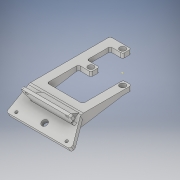
# Autodesk Inventor part: v3burnisher_cameras_mount
Saved by Autodesk Inventor 2019 (Build 230136000, 136)
## iProperties
Created: 2019-11-07
Part Number: v3burnisher_cameras_mount
Material: Generic
Document SubType Name: Modeling
Designer: luua
Density: 1 g/cm^3
Appearance: Default
Author: luua
Autodesk Inventor part; units mm, degrees
sketch "Sketch1" plane through (0, 0, 0) normal (0, 1, 0) x (-1, 0, 0)
  circle A0 centre (-17.6777, 17.6777) radius 3.3
  circle A1 centre (-17.6777, -17.6777) radius 3.25 construction
  circle A2 centre (17.6777, -17.6777) radius 3.3
  circle A3 centre (17.6777, 17.6777) radius 3.25 construction
  circle A4 centre (25, 0) radius 3 construction
  circle A5 centre (0, 0) radius 30.5 construction
  circle A6 centre (0, 0) radius 16.75 construction
  line L0 (36.4277, -22.4277) -> (12.9277, -22.4277)
  line L1 (12.9277, -22.4277) -> (12.9277, -12.9277)
  line L2 (12.9277, -12.9277) -> (26.9277, -12.9277)
  line L3 (26.9277, 57.5) -> (-12.9277, 57.5)
  line L4 (-12.9277, 57.5) -> (-12.9277, 12.3777)
  line L5 (-12.9277, 12.3777) -> (-22.4277, 12.3777)
  line L6 (-22.4277, 12.3777) -> (-22.4277, 67.5)
  line L7 (36.4277, -22.4277) -> (36.4277, 67.5)
  line L8 (32.5, 32.5) -> (-32.5, 32.5) construction
  line L9 (-32.5, 32.5) -> (-32.5, -32.5) construction
  line L10 (-32.5, -32.5) -> (32.5, -32.5) construction
  line L11 (32.5, -32.5) -> (32.5, 32.5) construction
  line L12 (32.5, 32.5) -> (-32.5, -32.5) construction
  line L13 (-32.5, 32.5) -> (32.5, -32.5) construction
  line L14 (20, 32.5) -> (20, 57.5) construction
  line L15 (20, 57.5) -> (-5, 57.5) construction
  line L16 (-5, 57.5) -> (-5, 32.5) construction
  line L17 (5, 57.5) -> (5, 32.5) construction
  line L18 (5, 32.5) -> (-5, 32.5) construction
  line L19 (36.4277, 67.5) -> (-22.4277, 67.5)
  line L20 (26.9277, -12.9277) -> (26.9277, 12.9277)
  line L21 (26.9277, 12.9277) -> (12.9277, 12.9277)
  line L22 (12.9277, 12.9277) -> (12.9277, 22.4277)
  line L23 (12.9277, 22.4277) -> (26.9277, 22.4277)
  circle A7 centre (17.6777, 17.6777) radius 3.25
  line L24 (26.9277, 22.4277) -> (26.9277, 57.5)
  point P0 (0, 32.5)
  point P1 (12.9277, -17.6777)
  point P2 (-17.6777, 12.3777)
  dimension "d0" = 65
  dimension "d1" = 65
  dimension "d2" = 10
  dimension "d3" = 15
  dimension "d4" = 25
  dimension "d5" = 2
  dimension "d7" = 4.75
  dimension "d8" = 4.75
  dimension "d9" = 4.75
  dimension "d96" = 6.6
  dimension "d97" = 6.6
  dimension "d99" = 4.75
  dimension "d100" = 4.75
  dimension "d101" = 9.5
  dimension "d102" = 14
  dimension "d103" = 9.5
  dimension "d104" = 10
  constraints: 50 end point, 10 perpendicular, 8 centre point, 6 midpoint, 5 point on line, 5 vertical, 4 horizontal, 2 collinear, 2 horizontal alignment, 2 parallel, 1 coincident, 1 concentric, 1 vertical alignment, 13 other
  measures "d0" distance of L10.end L9.end
  measures "d1" distance of L9.end L8.end
  measures "d2" distance between parallel lines of L16 L17
  measures "d3" distance between parallel lines of L14 L17
  measures "d4" distance of L15.end L16.end
  measures "d5" distance edge to line of A0 L5
  measures "d7" distance from line of A0.centre L4
  measures "d8" distance from line of L0 A2.centre
  measures "d9" distance from line of A2.centre L1
  measures "d96" diameter of A0
  measures "d97" diameter of A2
  measures "d99" distance from line of L22 A3.centre
  measures "d100" distance from line of L21 A3.centre
  measures "d101" distance between parallel lines of L23 L21
  measures "d102" distance of L1.end L2.end
  measures "d103" distance between parallel lines of L20 L7
  measures "d104" distance between parallel lines of L19 L15
extrude "Extrusion1" add sketch "Sketch1" along normal blind 5
ref_plane "Work Plane1" through (22.4277, 5, 67.5) normal (0, 0.8660254, 0.5) x (1, 0, 0)
sketch "Sketch4" plane through (22.4277, 5, 67.5) normal (0, 0.8660254, 0.5) x (1, 0, 0)
  line L0 (-58.8553, 0) -> (0, 0) projected
  line L1 (-23, 20) -> (-23, 0) construction
  circle A0 centre (-51, -25.748) radius 1.5
  circle A1 centre (5, -25.748) radius 1.5
  circle A2 centre (-23, -21.748) radius 3.25
  line L2 (-51, -25.748) -> (5, -25.748) construction
  line L3 (0, -2.5) -> (-58.8553, -2.5) projected
  line L4 (-58.8553, 77.8796) -> (-58.8553, 0) projected
  line L5 (-58.8553, -2.5) -> (-58.8553, 75.3796) projected
  line L6 (0, 45.2373) -> (0, -2.5) projected
  line L7 (0, 0) -> (0, -2.5)
  line L8 (0, -2.5) -> (12, -25.748)
  line L9 (12, -25.748) -> (12, -27.748)
  line L10 (-56.8553, -29.748) -> (10, -29.748)
  arc A3 (10, -29.748) -> (12, -27.748) centre (10, -27.748) ccw
  line L11 (-58.8553, -2.5) -> (-58.8553, -27.748)
  arc A4 (-58.8553, -27.748) -> (-56.8553, -29.748) centre (-56.8553, -27.748) ccw
  point P0 (-23, -25.748)
  point P1 (12, -29.748)
  dimension "d43" = 3
  dimension "d44" = 6.5
  dimension "d45" = 4
  dimension "d58" = 4
  dimension "d83" = 56
  dimension "d114" = 2
  constraints: 14 end point, 5 centre point, 4 point on circle, 4 tangent, 4 vertical, 3 point on line, 2 horizontal alignment, 2 vertical alignment, 1 coincident, 1 equal radius, 1 horizontal, 1 midpoint, 1 parallel, 1 perpendicular
  measures "d43" diameter of A0
  measures "d44" diameter of A2
  measures "d45" distance from line of L2 A2.centre
  measures "d58" distance from line of L10 L2.start
  measures "d83" distance of A1.centre L2.start
  measures "d114" radius of A4
extrude "Extrusion3" add sketch "Sketch4" against normal blind 5
sketch "Sketch5" plane through (22.4277, 5, 67.5) normal (0, 0.8660254, 0.5) x (1, 0, 0)
  line L0 (-45.5, -8.698) -> (-0.5, -8.698)
  line L1 (-0.5, -8.698) -> (-0.5, -11.698)
  line L2 (-0.5, -11.698) -> (-45.5, -11.698)
  line L3 (-45.5, -11.698) -> (-45.5, -8.698)
  line L4 (-58.8553, 0) -> (0, 0) projected
  line L5 (-58.8553, 0) -> (-58.8553, -27.748) projected
  line L6 (0, -2.5) -> (0, 0) projected
  line L7 (-56.8553, -29.748) -> (10, -29.748) projected
  line L8 (12, -27.748) -> (12, -25.748) projected
  line L9 (12, -25.748) -> (0, -2.5) projected
  arc A0 (10, -29.748) -> (12, -27.748) centre (10, -27.748) ccw projected
  circle A1 centre (-23, -21.748) radius 3.25 projected
  arc A2 (-58.8553, -27.748) -> (-56.8553, -29.748) centre (-56.8553, -27.748) ccw projected
  point P0 (-22.4277, 55.9567)
  point P1 (-23, -11.698)
  dimension "d50" = 3
  dimension "d51" = 45
  dimension "d62" = 10.05
  constraints: 8 end point, 2 parallel, 1 horizontal, 1 midpoint, 1 perpendicular, 1 vertical alignment
  measures "d50" distance of L0.end L1.end
  measures "d51" distance of L0.start L0.end
  measures "d62" distance from line of L2 A1.centre
extrude "Extrusion4" add sketch "Sketch5" along normal blind 4 contours L0 L1 L2 L3
sketch "Sketch7" plane through (22.4277, 8.4641, 69.5) normal (0, 0.8660254, 0.5) x (1, 0, 0)
  line L0 (-0.5, -8.698) -> (-45.5, -8.698) projected
  line L1 (-45.5, -8.698) -> (-45.5, -11.698) projected
  line L2 (-45.5, -11.698) -> (-0.5, -11.698) projected
  line L3 (-0.5, -11.698) -> (-0.5, -8.698) projected
  line L4 (-50.5, -11.698) -> (4.5, -11.698)
  line L5 (4.5, -11.698) -> (4.5, -8.698)
  line L6 (4.5, -8.698) -> (-50.5, -8.698)
  line L7 (-50.5, -8.698) -> (-50.5, -11.698)
  line L8 (-50.5, -11.698) -> (4.5, -8.698) construction
  line L9 (4.5, -11.698) -> (-50.5, -8.698) construction
  point P0 (-23, -10.198)
  dimension "d85" = 55
  constraints: 12 end point, 2 midpoint, 2 parallel, 1 horizontal, 1 perpendicular
  measures "d85" distance of L6.end L5.end
extrude "Extrusion5" add sketch "Sketch7" along normal blind 12
sketch "Sketch6" plane through (-23.0723, -0.849, 77.6307) normal (0, -0.5, 0.8660254) x (1, 0, 0)
  circle A0 centre (0, 12.5) radius 1.6
  circle A1 centre (45, 12.5) radius 1.6
  line L0 (45, 0) -> (0, 0) projected
  line L1 (45, 0) -> (45, 4) projected
  line L2 (0, 0) -> (0, 4) projected
  line L3 (0, 12.5) -> (45, 12.5) construction
  line L4 (45, 4) -> (50, 4) projected
  line L5 (50, 4) -> (50, 16) projected
  line L6 (-5, 16) -> (50, 16) projected
  line L7 (-5, 4) -> (-5, 16) projected
  line L8 (-5, 4) -> (0, 4) projected
  point P0 (22.5, 16)
  point P1 (22.5, 12.5)
  dimension "d67" = 12.5
  dimension "d74" = 3.2
  dimension "d75" = 3.2
  dimension "d84" = 45
  constraints: 2 centre point, 2 end point, 1 horizontal, 1 horizontal alignment, 1 midpoint, 1 vertical alignment
  measures "d67" distance from line of L0 L3.start
  measures "d74" diameter of A0
  measures "d75" diameter of A1
  measures "d84" distance of L3.end L3.start
extrude "Extrusion6" cut sketch "Sketch6" against normal up to next contours A0 | A1
sketch "Sketch8" plane through (-23.0723, -0.849, 77.6307) normal (0, -0.5, 0.8660254) x (1, 0, 0)
  line L0 (-5, 16) -> (50, 16) projected
  line L1 (22.5, 16) -> (22.5, 0) construction
  line L2 (-13.3553, 0) -> (45.5, 0) projected
  line L3 (0, 0) -> (0, 4) projected
  line L4 (0, 4) -> (-5, 4)
  line L5 (-5, 4) -> (-5, 9)
  line L6 (-5, 4) -> (-5, 16) projected
  line L7 (-5, 9) -> (0, 4)
  line L8 (45, 4) -> (50, 4)
  line L9 (50, 4) -> (50, 9)
  line L10 (50, 9) -> (45, 4)
  point P0 (23.0723, -38.0801)
  dimension "d86" = 5
  constraints: 14 end point, 3 symmetric about line, 2 point on line, 1 horizontal, 1 midpoint, 1 vertical
  measures "d86" distance of L4.end L5.end
extrude "Extrusion7" cut sketch "Sketch8" against normal up to surface (3 mm away)
ref_plane "Work Plane2" through (-0.5723, 14.5074, 83.0327) normal (-1, 0, 0) x (0, -0.5, 0.8660254)
sketch "Sketch9" plane through (-0.5723, 14.5074, 83.0327) normal (-1, 0, 0) x (0, -0.5, 0.8660254)
  line L0 (0, -6) -> (-8, -16)
  line L1 (-8, -16) -> (0, -16)
  line L2 (0, -16) -> (0, -6)
  point P0 (-64.6547, -54.0801)
  dimension "d88" = 10
  dimension "d89" = 8
  constraints: 6 end point, 1 horizontal, 1 perpendicular
  measures "d88" distance of L1.end L0.start
  measures "d89" distance of L0.end L1.end
extrude "Extrusion8" add sketch "Sketch9" along normal mid plane 40
ref_plane "Work Plane3" through (-7, 0, 12.3777) normal (1, 0, 0) x (0, 0, -1)
sketch "Sketch10" plane through (-7, 0, 12.3777) normal (1, 0, 0) x (0, 0, -1)
  line L0 (-70.3848, -9.5853) -> (-10.05, 0)
  line L1 (0, 0) -> (-53.7826, 0) projected
  line L2 (-70.3848, -9.5853) -> (-53.7826, 0)
  line L3 (-53.7826, 0) -> (-10.05, 0)
  line L4 (-68.642, -8.5791) -> (-74.2712, -11.8291) projected
  point P0 (-78.3848, -14.2041)
  dimension "d115" = 8
  constraints: 6 end point, 2 point on line, 1 coincident, 1 collinear
  measures "d115" horizontal distance of point (-78.385, -14.204) L0.start
extrude "Extrusion11" add sketch "Sketch10" along normal blind 9.5 from surface at -29.4277
extrude "Extrusion12" add sketch "Sketch10" along normal blind 9.5 from surface at 19.9277
sketch "Sketch12" plane through (12.9277, 0, 57.5) normal (-1, 0, 0) x (0, 0, 1)
  line L0 (8.6603, 0) -> (25.2625, -9.5853) projected
  line L1 (0, 0) -> (0, 5) projected
  line L2 (8.6603, 0) -> (0, 0)
  line L3 (8.6603, 0) -> (25.2625, -9.5853)
  line L4 (32.2984, -7.874) -> (12.1651, 3.75) projected
  line L5 (25.2625, -9.5853) -> (-35.0723, 0) projected
  line L6 (25.2625, -9.5853) -> (0, -5.5719)
  line L7 (0, 0) -> (0, -5.5719)
  point P0 (-57.5, 0)
  constraints: 8 end point, 1 horizontal, 1 parallel, 1 point on line, 1 vertical
extrude "Extrusion13" add sketch "Sketch12" along normal up to next
fillet "Fillet3" [suppressed]
sketch "Sketch13" plane through (22.4277, 0.6699, 65) normal (0, -0.8660254, -0.5) x (1, 0, 0)
  arc A0 (-19.9949, 20.5104) -> (-26.0051, 20.5104) centre (-23, 21.748) ccw projected
  arc A1 (-26.0051, 20.5104) -> (-19.9949, 20.5104) centre (-23, 21.748) ccw projected
  circle A2 centre (-23, 21.748) radius 7.5
  point P0 (-22.4277, -55.9567)
  dimension "d118" = 15
  constraints: 1 centre point, 1 coincident
  measures "d118" diameter of A2
extrude "Extrusion14" cut sketch "Sketch13" along normal blind 10 contours A1 A0
extrude "Extrusion15" cut sketch "Sketch13" along normal blind 5
fillet "Fillet4" radius 2 8 edges at (26.9277, 7.6952, 80.8317) (-28.0723, 7.6952, 80.8317) (-28.0723, 13.7574, 84.3317) (-23.0723, -0.099, 76.3317) (21.9277, -0.099, 76.3317) (26.9277, 13.7574, 84.3317) (-23.0723, 3.3651, 78.3317) (21.9277, 3.3651, 78.3317)
fillet "Fillet4" radius 5 1 edges at (-7, 5, 67.5)
fillet "Fillet4" radius 2 12 edges at (-26.9277, 2.5, 22.4277) (-26.9277, 2.5, 12.9277) (-26.9277, 2.5, -12.9277) (-12.9277, 2.5, -22.4277) (-12.9277, 2.5, -12.9277) (-12.9277, 2.5, 12.9277) (-12.9277, 2.5, 22.4277) (22.4277, 2.5, 12.3777) (12.9277, 2.5, 12.3777) (-36.4277, 2.5, -22.4277) (-26.9277, -0.2859, 57.5) (12.9277, -0.2859, 57.5)
equation "\"d8\" = d7"
equation "\"d9\" = d8"
equation "\"d75\" = d74"
body "Solid1"
